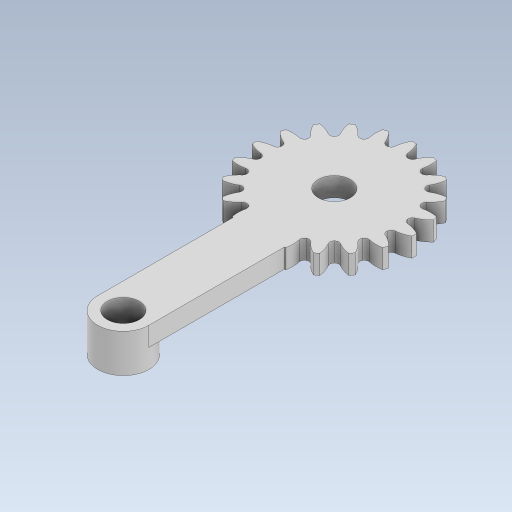
# Autodesk Inventor part: Gear Link
Saved by Autodesk Inventor 2023.5 (Build 275446000, 446)
## iProperties
Created: 2025-10-05
Part Number: Gear Link
Material: Generic
Document SubType Name: Modeling
Designer: Guntur
Density: 1 g/cm^3
Appearance: Default
Mass: 1.04129 g
Surface Area: 14.3231 cm^2
Volume: 1.04129 cm^3
Author: Guntur
## iProperties of the stored document Gear Link_3DPrint.ipt
Created: 2025-10-05
Part Number: Gear Link_3DPrint
Material: Generic
Document SubType Name: Modeling
Designer: Guntur
Density: 1 g/cm^3
Appearance: Default
Author: Guntur
Autodesk Inventor part; units mm, degrees
ref_plane "YZ Plane" through (0, 0, 0) normal (1, 0, 0) x (0, 1, 0)
ref_plane "XZ Plane" through (0, 0, 0) normal (0, 1, 0) x (-1, 0, 0)
ref_plane "XY Plane" through (0, 0, 0) normal (0, 0, 1) x (1, 0, 0)
sketch "Sketch1" plane through (0, 0, 0) normal (0, 1, 0) x (-1, 0, 0)
  circle A0 centre (0, 0) radius 10
  line L0 (14.2875, 0) -> (-14.2875, 0) construction
  line L1 (0, 15.875) -> (0, -15.875) construction
  circle A1 centre (0, 0) radius 12.5
  circle A2 centre (0, 0) radius 11.5
  arc A3 (12.4951, 0.35) -> (9.9499, 1) centre (10.0249, -4.0143) ccw
  arc A4 (9.9499, -1) -> (12.4951, -0.35) centre (10.0249, 4.0143) ccw
  circle A5 centre (0, 0) radius 2.5
  point P0 (9.9499, -1)
  point P1 (12.4951, -0.35)
  dimension "d0" = 20
  dimension "d1" = 25
  dimension "d2" = 23
  dimension "d3" = 2
  dimension "d4" = 0.7
  dimension "d15" = 5
  constraints: 4 centre point, 4 coincident, 4 end point, 4 point on circle, 3 symmetric about line, 1 horizontal, 1 vertical, 7 other
  measures "d2" diameter of A2
  measures "d3" distance of A4.start A3.end
  measures "d4" distance of A4.end A3.start
  measures "d15" diameter of A5
extrude "Extrusion1" add sketch "Sketch1" along normal blind 3 contours A0
extrude "Extrusion3" add sketch "Sketch1" along normal blind 3 contours A0 A3 A2 A4 | A3 A1 A4 A2 picked at (10.8217, 0.5021) picked at (12.0552, 0.1736)
fillet "Fillet1" radius 0.7 2 edges at (-9.9499, 1.5, 1) (-9.9499, 1.5, -1)
pattern_circular "Circular Pattern1" count 20 over 360 about axis through (0, 0, 0) along (0, 1, 0) of "Fillet1", "Extrusion3"
ref_plane "Work Plane1" through (0, 1.5, 0) normal (0, 1, 0) x (1, 0, 0)
sketch "Sketch2" plane through (0, 1.5, 0) normal (0, 1, 0) x (1, 0, 0)
  circle A0 centre (0, -33) radius 4
  line L0 (4, -33) -> (4, -3)
  line L1 (-4, -33) -> (-4, -3)
  line L2 (4, -3) -> (-4, -3)
  circle A1 centre (0, 0) radius 3.5
  circle A2 centre (0, -33) radius 2.5
  point P0 (3.5, 0)
  point P1 (-3.5, 0)
  dimension "d16" = 8
  dimension "d17" = 33
  dimension "d18" = 7
  dimension "d19" = 5
  constraints: 6 end point, 3 centre point, 2 coincident, 2 point on circle, 2 vertical, 1 horizontal
  measures "d16" diameter of A0
  measures "d17" distance of A0.centre point (0, 0)
  measures "d18" diameter of A1
  measures "d19" diameter of A2
extrude "Extrusion4" add sketch "Sketch2" along normal mid plane 3 contours A0 | A0 L1 L2 A1 L0 | A1 L2 picked at (-0.3722, -3.1057)
extrude "Extrusion5" add sketch "Sketch2" against normal blind 4.5 contours A0
body "Solid1"
